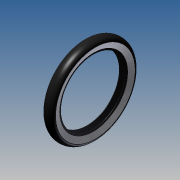
# Autodesk Inventor part: pneu
Saved by Autodesk Inventor 2014 SP1 (Build 180222100, 222)
## iProperties
Created: 2012-06-12
Part Number: pneu
Material: Plastique ABS
Document SubType Name: Modeling
Designer: Luis
Density: 1.06 g/cm^3
Appearance: Lustré - Noir
d17: 35,000 mm
d19: 15,000 mm
d29: 45,00 deg
d31: 5,000 mm
d32: 0,00 deg
d33: 20,000 nd
d34: 360,00 deg
d44: 12,000 mm
d59: 3,000 mm
Author: Luis
Autodesk Inventor part; units mm, degrees
ref_plane "YZ Plane" through (0, 0, 0) normal (1, 0, 0) x (0, 1, 0)
ref_plane "XZ Plane" through (0, 0, 0) normal (0, 1, 0) x (-1, 0, 0)
ref_plane "XY Plane" through (0, 0, 0) normal (0, 0, 1) x (1, 0, 0)
sketch "Sketch1" plane through (0, 0, 0) normal (0, 0, 1) x (1, 0, 0)
  line L0 (34, 248.5307) -> (23.32, 215.2)
  line L1 (23.32, 215.2) -> (20.32, 215.2)
  line L2 (20.32, 215.2) -> (20.32, 203.2)
  line L3 (17.32, 203.2) -> (20.32, 203.2)
  line L4 (17.32, 203.2) -> (17.32, 220.2)
  line L5 (17.32, 220.2) -> (20.32, 220.2)
  line L6 (20.32, 220.2) -> (20.32, 248.5307)
  line L7 (-82.1062, 0) -> (56.8109, 0) projected
  line L8 (0, 344.4318) -> (0, -57.4053) construction
  line L9 (-20.32, 248.5307) -> (-28.3333, 264.7913) construction
  line L10 (-28.3333, 264.7913) -> (0, 268.1013) construction
  line L11 (0, 268.1013) -> (28.3333, 264.7913) construction
  line L12 (28.3333, 264.7913) -> (20.32, 248.5307) construction
  spline S0 degree 4 poles (-20.32, 248.5307) (-28.3333, 264.7913) (0, 268.1013) (28.3333, 264.7913) (20.32, 248.5307) knots 1 1 1 1 1 2 2 2 2 2
  line L13 (-34, 248.5307) -> (-23.32, 215.2)
  line L14 (-23.32, 215.2) -> (-20.32, 215.2)
  line L15 (-20.32, 215.2) -> (-20.32, 203.2)
  line L16 (-17.32, 203.2) -> (-20.32, 203.2)
  line L17 (-17.32, 203.2) -> (-17.32, 220.2)
  line L18 (-17.32, 220.2) -> (-20.32, 220.2)
  line L19 (-20.32, 220.2) -> (-20.32, 248.5307)
  line L20 (20.32, 248.5307) -> (34, 248.5307) construction
  line L21 (-34, 248.5307) -> (34, 248.5307) construction
  line L22 (34, 248.5307) -> (36.9656, 270.5975) construction
  line L23 (36.9656, 270.5975) -> (0, 287.0265) construction
  line L24 (0, 287.0265) -> (-36.9656, 270.5975) construction
  line L25 (-36.9656, 270.5975) -> (-34, 248.5307) construction
  spline S1 degree 4 poles (34, 248.5307) (36.9656, 270.5975) (0, 287.0265) (-36.9656, 270.5975) (-34, 248.5307) knots 1 1 1 1 1 2 2 2 2 2
  point P0 (0, 0)
  point P1 (0, 0)
  point P2 (0, 0)
  point P3 (0, 264)
  point P4 (0, 274)
  dimension "d17" = 35
  dimension "d44" = 12
  dimension "d59" = 3
  dimension "d64" = 10
  dimension "d66" = 274
  dimension "d67" = 68
  dimension "d68" = 40.64
  dimension "d69" = 203.2
  dimension "d70" = 5
  constraints: 32 end point, 9 symmetric about line, 4 perpendicular, 4 point on line, 2 parallel, 1 coincident, 1 collinear, 10 other
  measures "d17" distance of L0.end L0.start
  measures "d44" distance between parallel lines of L1 L3
  measures "d59" distance between parallel lines of L2 L4
  measures "d64" distance of point (0, 274) point (0, 264)
  measures "d66" distance from line of L7 point (0, 274)
  measures "d67" distance of L0.start L13.start
  measures "d68" distance between parallel lines of L15 L2
  measures "d69" distance between parallel lines of L3 L7
  measures "d70" distance between parallel lines of L1 L5
revolve "Revolution1" add sketch "Sketch1" angle 360 about axis through (-10, 0, 0) along (1, 0, 0)
sketch "Sketch3" plane through (0, 0, 0) normal (0, 1, 0) x (-1, 0, 0)
  line L0 (0, 0) -> (0, 77.3111)
  line L1 (0, 0) -> (62.2609, 62.2609)
  dimension "d29" = 45
  constraints: 4 end point, 1 vertical
  measures "d29" angle of L1 L0
ref_plane "Work Plane1" through (0, 0, 0) normal (-0.7071068, 0, 0.7071068) x (0, -1, 0)
sketch "Sketch4" plane through (0, 0, 0) normal (-0.7071068, 0, 0.7071068) x (0, -1, 0)
  line L0 (0, -290.7432) -> (0, 290.7432) projected
  line L1 (399.5747, 0) -> (-404.7199, 0) construction
  ellipse E0 centre (0, 19.0919) end of major axis (-266.695, 19.0919) minor radius 188.5818 construction
  ellipse E1 centre (0, -19.0919) end of major axis (-266.695, -19.0919) minor radius 188.5818 construction
  line L2 (-265.3248, 38.1838) -> (-247.0972, 38.1838) construction
  line L3 (-247.225, -38.1838) -> (-265.3248, -38.1838) construction
  ellipse E2 centre (0, 0) end of major axis (0, 357.3647) minor radius 252.695 (-251.8209, -29.6985) -> (-251.5527, -33.9411) ccw construction
  line L4 (-264.8083, -33.9411) -> (-251.5527, -33.9411) construction
  line L5 (-251.5527, 33.9411) -> (-264.8083, 33.9411) construction
  ellipse E3 centre (0, 0) end of major axis (0, 357.3647) minor radius 252.695 (-251.5527, 33.9411) -> (-251.8209, 29.6985) ccw construction
  line L6 (-238.5043, 29.6985) -> (-251.8209, 29.6985) construction
  line L7 (-243.5152, 33.9411) -> (-238.4904, 33.9411) construction
  line L8 (238.4904, 33.9411) -> (243.5152, 33.9411) projected
  line L9 (251.8209, 29.6985) -> (238.5043, 29.6985) projected
  ellipse E4 centre (0, 0) end of major axis (0, 357.3647) minor radius 252.695 (251.8209, 29.6985) -> (251.5527, 33.9411) ccw projected
  line L10 (264.8083, 33.9411) -> (251.5527, 33.9411) projected
  line L11 (251.5527, -33.9411) -> (264.8083, -33.9411) projected
  ellipse E5 centre (0, 0) end of major axis (0, 357.3647) minor radius 252.695 (251.5527, -33.9411) -> (251.8209, -29.6985) ccw projected
  line L12 (265.3248, -38.1838) -> (247.225, -38.1838) projected
  line L13 (247.0972, 38.1838) -> (265.3248, 38.1838) projected
  line L14 (-251.8209, -29.6985) -> (-246.5751, -29.6985) construction
  line L15 (246.5751, -29.6985) -> (251.8209, -29.6985) projected
  line L16 (-277.5443, 14.9358) -> (-262.8286, 59.481)
  line L17 (-262.8286, 59.481) -> (-270.0708, 46.2329)
  line L18 (-270.0708, 46.2329) -> (-267.1666, 35.1533)
  line L19 (-267.1666, 35.1533) -> (-265.2666, 33.5992)
  constraints: 8 end point, 3 vertical alignment, 29 other
body "Solid1"
